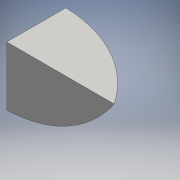
# Autodesk Inventor part: corner_insert
Saved by Autodesk Inventor 2016 (Build 200138000, 138)
## iProperties
Created: 2018-03-11
Part Number: corner_insert
Material: Generic
Document SubType Name: Modeling
Designer: Mick
Density: 1 g/cm^3
Appearance: Default
Author: Mick
Autodesk Inventor part; units mm, degrees
ref_plane "YZ Plane" through (0, 0, 0) normal (1, 0, 0) x (0, 1, 0)
ref_plane "XZ Plane" through (0, 0, 0) normal (0, 1, 0) x (-1, 0, 0)
ref_plane "XY Plane" through (0, 0, 0) normal (0, 0, 1) x (1, 0, 0)
sketch "Sketch1" plane through (0, 0, 0) normal (0, 1, 0) x (-1, 0, 0)
  arc A0 (-1.1282, -10.942) -> (0, -11) centre (0, 0) ccw
  line L0 (0, 0) -> (0, -11)
  line L1 (0, 0) -> (-11, 0)
  line L2 (0, 0) -> (-20, 0)
  arc A1 (-20, 0) -> (0, -11) centre (0.7193, 13.9896) ccw
  dimension "d4" = 22
  dimension "d15" = 20
  dimension "d16" = 25
  constraints: 6 end point, 5 point on circle, 2 centre point, 2 horizontal, 1 coincident, 1 point on line
  measures "d4" diameter of A0
  measures "d15" distance of L0.start L2.end
  measures "d16" radius of A1
revolve "Revolution1" add sketch "Sketch1" angle 90 about axis through (0, 0, 0) along (1, 0, 0) contours A1 L2 L1 L0
sketch "Sketch2" plane through (0, 0, -11) normal (-1, 0, 0) x (0, 0, 1)
  line L0 (11, 0) -> (3.2218, 7.7782)
  arc A0 (11, 11) -> (0, 0) centre (11, 0) ccw projected
  line L1 (11, 11) -> (11, 0) projected
  point P0 (6, 5)
  dimension "d6" = 45
  dimension "d7" = 5
  constraints: 2 end point, 1 point on circle, 1 point on line
  measures "d6" angle of L0 L1
  measures "d7" horizontal distance of point (6, 5) L0.start
hole "Hole1" at (0, 5, -5) direction (1, 0, 0) diameter 4 depth 8 tip angle 118
body "Solid1"
